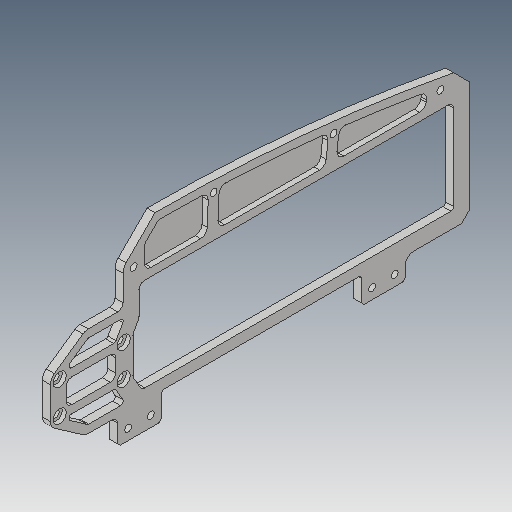
# Autodesk Inventor part: VerticalFrame
Saved by Autodesk Inventor 2019.4 (Build 234330000, 330)
## iProperties
Created: 2019-01-12
Part Number: VerticalFrame
Material: 一般
Document SubType Name: Modeling
Designer: y6tada
Density: 1 g/cm^3
Appearance: 既定
Mass: 8.8829 g
Surface Area: 108.713 cm^2
Volume: 8.8829 cm^3
Author: y6tada
Autodesk Inventor part; units mm, degrees
ref_plane "YZ Plane" through (0, 0, 0) normal (1, 0, 0) x (0, 1, 0)
ref_plane "XZ Plane" through (0, 0, 0) normal (0, 1, 0) x (-1, 0, 0)
ref_plane "XY Plane" through (0, 0, 0) normal (0, 0, 1) x (1, 0, 0)
sketch "スケッチ1" plane through (0, 0, 0) normal (1, 0, 0) x (0, 1, 0)
  line L0 (32.2256, 59) -> (0.2256, 59) construction
  line L1 (-0.7744, 56.7973) -> (-0.7744, -58)
  line L2 (0.2256, -59) -> (32.2256, -59)
  line L3 (34.2256, -57) -> (34.2256, 57)
  line L4 (-7, 67.0882) -> (-13.7744, 67.0882)
  line L5 (-14.7744, 66.0882) -> (-14.7744, 51.5882)
  line L6 (-13.7744, 50.5882) -> (-5.7744, 50.5882)
  line L7 (-4.7744, 49.5882) -> (-4.7744, -23.4118)
  line L8 (-5.7744, -24.4118) -> (-13.7744, -24.4118)
  line L9 (-14.7744, -25.4118) -> (-14.7744, -39.9118)
  line L10 (-13.7744, -40.9118) -> (-9.7744, -40.9118)
  line L11 (-3.7744, -65) -> (37.6795, -65)
  line L12 (18, 92.25) -> (6, 92.25)
  line L13 (0, 0) -> (34.2256, 0) construction
  line L14 (-6.7744, -62) -> (-3.7744, -65)
  line L15 (31, 65) -> (40.5687, 65)
  circle A0 centre (-10.7744, 63.0882) radius 1.3
  circle A1 centre (-10.7744, 54.5882) radius 1.3
  circle A2 centre (-10.7744, -28.4118) radius 1.3
  circle A3 centre (-10.7744, -36.9118) radius 1.3
  line L16 (-10.7744, 63.0882) -> (-10.7744, 54.5882) construction
  circle A4 centre (-10.7744, 63.0882) radius 2 construction
  circle A5 centre (-10.7744, 54.5882) radius 2 construction
  line L17 (-10.7744, -28.4118) -> (-10.7744, -36.9118) construction
  circle A6 centre (18, 88.75) radius 1.05 construction
  circle A7 centre (6, 88.75) radius 1.05 construction
  circle A8 centre (6, 64.75) radius 1.05 construction
  circle A9 centre (18, 64.75) radius 1.05 construction
  circle A10 centre (18, 88.75) radius 1.3
  circle A11 centre (6, 88.75) radius 1.3
  circle A12 centre (6, 64.75) radius 1.3
  circle A13 centre (18, 64.75) radius 1.3
  arc A14 (20.867, 90.7575) -> (18, 92.25) centre (18, 88.75) ccw
  arc A15 (6, 92.25) -> (3.133, 90.7575) centre (6, 88.75) ccw
  line L18 (-6.7744, -43.9118) -> (-6.7744, -62)
  arc A16 (-6.7744, -43.9118) -> (-9.7744, -40.9118) centre (-9.7744, -43.9118) ccw
  arc A17 (34.2256, 57) -> (32.2256, 59) centre (32.2256, 57) ccw
  arc A18 (32.2256, -59) -> (34.2256, -57) centre (32.2256, -57) ccw
  line L19 (43.3971, 63.8284) -> (54.2256, 53)
  arc A19 (43.6795, -59) -> (54.2256, 53) centre (-545.7744, 53) ccw
  line L20 (54.2256, 80.46) -> (54.2256, 17.89) construction
  arc A20 (-0.7744, -58) -> (0.2256, -59) centre (0.2256, -58) ccw
  arc A21 (43.3971, 63.8284) -> (40.5687, 65) centre (40.5687, 61) ccw
  line L21 (20.867, 90.7575) -> (28.367, 80.0464)
  line L22 (29, 78.0389) -> (29, 67)
  line L23 (3.133, 90.7575) -> (-4.367, 80.0464)
  line L24 (-5, 78.0389) -> (-5, 69.0882)
  line L25 (12, 92.25) -> (12, 64.3882) construction
  arc A22 (29, 78.0389) -> (28.367, 80.0464) centre (25.5, 78.0389) ccw
  arc A23 (-4.367, 80.0464) -> (-5, 78.0389) centre (-1.5, 78.0389) ccw
  arc A24 (29, 67) -> (31, 65) centre (31, 67) ccw
  arc A25 (-7, 67.0882) -> (-5, 69.0882) centre (-7, 69.0882) ccw
  line L26 (14.5, 86.25) -> (9.5, 86.25)
  line L27 (7.5, 84.25) -> (7.5, 69.75)
  line L28 (9.5, 67.75) -> (14.5, 67.75)
  line L29 (16.5, 69.75) -> (16.5, 84.25)
  arc A26 (16.5, 84.25) -> (14.5, 86.25) centre (14.5, 84.25) ccw
  arc A27 (14.5, 67.75) -> (16.5, 69.75) centre (14.5, 69.75) ccw
  arc A28 (7.5, 69.75) -> (9.5, 67.75) centre (9.5, 69.75) ccw
  arc A29 (9.5, 86.25) -> (7.5, 84.25) centre (9.5, 84.25) ccw
  line L30 (19.5, 84.3079) -> (19.5, 68.5028)
  line L31 (20, 67.6368) -> (24.5, 65.0387)
  line L32 (26, 65.9047) -> (26, 77.8812)
  line L33 (25.8192, 78.4548) -> (21.3192, 84.8815)
  arc A30 (24.5, 65.0387) -> (26, 65.9047) centre (25, 65.9047) ccw
  arc A31 (19.5, 68.5028) -> (20, 67.6368) centre (20.5, 68.5028) ccw
  arc A32 (21.3192, 84.8815) -> (19.5, 84.3079) centre (20.5, 84.3079) ccw
  arc A33 (26, 77.8812) -> (25.8192, 78.4548) centre (25, 77.8812) ccw
  line L34 (4.5, 84.3079) -> (4.5, 68.5028)
  line L35 (4, 67.6368) -> (-0.5, 65.0387)
  line L36 (-2, 65.9047) -> (-2, 77.8812)
  line L37 (-1.8192, 78.4548) -> (2.6808, 84.8815)
  arc A34 (-2, 65.9047) -> (-0.5, 65.0387) centre (-1, 65.9047) ccw
  arc A35 (4, 67.6368) -> (4.5, 68.5028) centre (3.5, 68.5028) ccw
  arc A36 (4.5, 84.3079) -> (2.6808, 84.8815) centre (3.5, 84.3079) ccw
  arc A37 (-1.8192, 78.4548) -> (-2, 77.8812) centre (-1, 77.8812) ccw
  arc A38 (-4.7744, 49.5882) -> (-5.7744, 50.5882) centre (-5.7744, 49.5882) ccw
  arc A39 (-5.7744, -24.4118) -> (-4.7744, -23.4118) centre (-5.7744, -23.4118) ccw
  line L38 (-13.7744, 67.0882) -> (-14.7744, 66.0882)
  line L39 (-14.7744, 51.5882) -> (-13.7744, 50.5882)
  line L40 (-13.7744, -24.4118) -> (-14.7744, -25.4118)
  line L41 (-14.7744, -39.9118) -> (-13.7744, -40.9118)
  circle A40 centre (40.5687, 61) radius 1.3
  line L42 (54.2256, 53) -> (-545.7744, 53) construction
  line L43 (37.6795, -65) -> (43.6795, -59)
  arc A41 (39.7277, -58.3699) -> (50.2221, 55.0291) centre (-545.7744, 53) ccw construction
  circle A42 centre (49.8194, 31) radius 1.3
  circle A43 centre (46.4476, -14) radius 1.3
  circle A44 centre (40.542, -54) radius 1.3
  line L44 (22.4952, 59.2679) -> (19.5263, 60.9821)
  line L45 (18.5263, 61.25) -> (5.4737, 61.25)
  line L46 (4.4737, 60.9821) -> (0.2256, 58.5294)
  line L47 (32.2256, 59) -> (23.4952, 59)
  arc A45 (22.4952, 59.2679) -> (23.4952, 59) centre (23.4952, 61) ccw
  arc A46 (19.5263, 60.9821) -> (18.5263, 61.25) centre (18.5263, 59.25) ccw
  arc A47 (5.4737, 61.25) -> (4.4737, 60.9821) centre (5.4737, 59.25) ccw
  arc A48 (0.2256, 58.5294) -> (-0.7744, 56.7973) centre (1.2256, 56.7973) ccw
  point P0 (34.2256, 59)
  point P1 (-0.7744, -59)
  point P2 (-0.7744, 59)
  point P3 (34.2256, -59)
  point P4 (-10.0245, 67.0882)
  point P5 (-14.7744, 67.0882)
  point P6 (-14.7744, 50.5882)
  point P7 (-4.7744, 50.5882)
  point P8 (-4.7744, -24.4118)
  point P9 (-14.7744, -24.4118)
  point P10 (-14.7744, -40.9118)
  point P11 (-4.7744, -40.9118)
  point P12 (2.5, 68.5585)
  point P13 (42.2256, 65)
  point P14 (24.5, 65)
  point P15 (-0.5, 67.0882)
  point P16 (-0.7744, 58)
  point P17 (-1.5, 78.0389)
  point P18 (22.9593, 59)
  dimension "d2" = 118
  dimension "d4" = 108
  dimension "d5" = 16.5
  dimension "d6" = 16.5
  dimension "d7" = 4
  dimension "d8" = 2.6
  dimension "d10" = 4
  dimension "d11" = 4
  dimension "d12" = 4
  dimension "d13" = 4
  dimension "d14" = 4
  dimension "d15" = 4
  dimension "d16" = 10
  dimension "d17" = 2.6
  dimension "d18" = 3.5
  dimension "d20" = 35
  dimension "d21" = 3
  dimension "d22" = 6
  dimension "d24" = 2
  dimension "d26" = 45
  dimension "d27" = 600
  dimension "d28" = 20
  dimension "d29" = 6
  dimension "d30" = 45
  dimension "d32" = 3
  dimension "d33" = 1
  dimension "d36" = 4
  dimension "d37" = 35
  dimension "d38" = 35
  dimension "d39" = 34
  dimension "d40" = 3.5
  dimension "d41" = 2
  dimension "d42" = 6
  dimension "d43" = 3
  dimension "d44" = 9
  dimension "d45" = 2
  dimension "d46" = 1
  dimension "d47" = 3
  dimension "d48" = 3
  dimension "d49" = 3
  dimension "d50" = 3.5
  dimension "d51" = 1
  dimension "d52" = 1
  dimension "d53" = 45
  dimension "d54" = 1
  dimension "d55" = 45
  dimension "d56" = 1
  dimension "d57" = 45
  dimension "d58" = 1
  dimension "d59" = 45
  dimension "d60" = 45
  dimension "d61" = 6
  dimension "d62" = 4
  dimension "d63" = 30
  dimension "d64" = 45
  dimension "d65" = 40
  dimension "d69" = 120
  dimension "d70" = 6
  dimension "d71" = 6.5
  dimension "d72" = 6
  dimension "d73" = 6
  dimension "d74" = 2
  dimension "d93" = 12
  constraints: 96 end point, 65 point on circle, 51 tangent, 43 centre point, 31 point on line, 24 equal radius, 13 symmetric about line, 10 parallel, 9 perpendicular, 7 vertical, 6 horizontal, 5 coincident, 3 concentric, 2 collinear, 2 midpoint, 6 other
  measures "d2" distance of point (34.226, -59) point (34.226, 59)
  measures "d4" distance between parallel lines of L4 L10
  measures "d5" distance of point (-14.774, -24.412) point (-14.774, -40.912)
  measures "d6" distance of point (-14.774, 67.088) point (-14.774, 50.588)
  measures "d7" distance from line of L17.start L8
  measures "d8" diameter of A2
  measures "d10" distance from line of L10 L17.end
  measures "d11" distance between parallel lines of L5 L16
  measures "d12" distance from line of L6 L16.end
  measures "d13" distance from line of L4 L16.start
  measures "d14" distance between parallel lines of L17 L9
  measures "d15" distance between parallel lines of L1 L7
  measures "d16" distance of point (-14.774, 50.588) point (-4.774, 50.588)
  measures "d17" diameter of A10
  measures "d18" radius of A14
  measures "d20" distance of point (34.226, 59) point (-0.774, 59)
  measures "d21" radius of A16
  measures "d22" distance between parallel lines of L18 L1
  measures "d24" radius of A17
  measures "d26" angle of L19 L15
  measures "d27" radius of A19
  measures "d28" distance between parallel lines of L3 L20
  measures "d29" distance between parallel lines of L11 L2
  measures "d30" angle of L14 L18
  measures "d32" distance from line of L14.start L11
  measures "d33" radius of A20
  measures "d36" radius of A21
  measures "d37" angle of L22 L21
  measures "d38" angle of L24 L23
  measures "d39" distance between parallel lines of L24 L22
  measures "d40" radius of A22
  measures "d41" radius of A24
  measures "d42" distance between parallel lines of L26 L12
  measures "d43" distance from line of A9.centre L28
  measures "d44" distance between parallel lines of L27 L29
  measures "d45" radius of A26
  measures "d46" radius of A30
  measures "d47" distance between parallel lines of L22 L32
  measures "d48" distance between parallel lines of L21 L33
  measures "d49" distance between parallel lines of L29 L30
  measures "d50" distance from line of A9.centre L31
  measures "d51" radius of A38
  measures "d52" distance of L4.end point (-14.774, 67.088)
  measures "d53" angle of L4 L38
  measures "d54" distance of L5.end point (-14.774, 50.588)
  measures "d55" angle of L5 L39
  measures "d56" distance of L8.end point (-14.774, -24.412)
  measures "d57" angle of L8 L40
  measures "d58" distance of L9.end point (-14.774, -40.912)
  measures "d59" angle of L9 L41
  measures "d60" angle of L43 L11
  measures "d61" distance from line of L43.end L11
  measures "d62" radial gap between concentric circles of A41 A19
  measures "d63" vertical distance of A42.centre A21.centre
  measures "d64" vertical distance of A43.centre A42.centre
  measures "d65" vertical distance of A44.centre A43.centre
  measures "d69" angle of L30 L31
  measures "d70" distance between parallel lines of L0 L15
  measures "d71" distance between parallel lines of L28 L45
  measures "d72" distance between parallel lines of L31 L44
  measures "d73" distance between parallel lines of L35 L46
  measures "d74" radius of A45
  measures "d93" distance between parallel lines of L42 L15
extrude "押し出し1" add sketch "スケッチ1" along normal blind 3
sketch "スケッチ2" plane through (3, 0, 0) normal (1, 0, 0) x (0, 0, -1)
  circle A0 centre (-88.75, 18) radius 1.3 projected
  circle A1 centre (-88.75, 18) radius 2.5
  circle A2 centre (-88.75, 6) radius 1.3 projected
  circle A3 centre (-88.75, 6) radius 2.5
  circle A4 centre (-64.75, 6) radius 1.3 projected
  circle A5 centre (-64.75, 6) radius 2.5
  circle A6 centre (-64.75, 18) radius 1.3 projected
  circle A7 centre (-64.75, 18) radius 2.5
  point P0 (0, 0)
  dimension "d66" = 5
  constraints: 4 centre point, 4 coincident, 3 equal radius
  measures "d66" diameter of A1
extrude "押し出し2" cut sketch "スケッチ2" against normal blind 1.5
sketch "スケッチ3" plane through (3, 0, 0) normal (1, 0, 0) x (0, 0, -1)
  circle A0 centre (-31, 49.8194) radius 1.3 construction
  line L0 (-31, 49.8194) -> (-31.9952, 22.8769) construction
  circle A1 centre (14, 46.4476) radius 1.3 construction
  line L1 (14, 46.4476) -> (11.2386, 22.0394) construction
  arc A2 (11.2386, 22.0394) -> (11.2386, 22.0394) centre (23.9128, 20.6055) ccw
  line L2 (-53, 54.2256) -> (-63.8284, 43.3971) construction
  arc A3 (59, 43.6795) -> (-53, 54.2256) centre (-53, -545.7744) ccw construction
  line L3 (-57, 34.2256) -> (57, 34.2256) construction
  line L4 (-52.4939, 50.489) -> (-56.2678, 46.7152)
  line L5 (-33.0546, 48.3772) -> (-33.3776, 39.6333)
  line L6 (-29.0574, 48.2296) -> (-29.3681, 39.8178)
  line L7 (-57, 39.7256) -> (-57, 44.9474)
  line L8 (11.8421, 45.1651) -> (11.195, 39.4445)
  line L9 (15.8168, 44.7154) -> (15.2841, 40.0066)
  circle A4 centre (54, 40.542) radius 1.3 construction
  line L10 (54, 40.542) -> (51.075, 24.5141) construction
  line L11 (48.8034, 39.9175) -> (48.6865, 39.2767)
  line L12 (-54.5, 37.2256) -> (-35.8759, 37.2256)
  line L13 (-26.8698, 37.2256) -> (8.7108, 37.2256)
  line L14 (17.7682, 37.2256) -> (46.2271, 37.2256)
  arc A5 (-35.4796, 50.9684) -> (-50.7166, 51.2212) centre (-53, -545.7744) ccw
  arc A6 (-50.7166, 51.2212) -> (-52.4939, 50.489) centre (-50.7262, 48.7212) ccw
  arc A7 (-33.0546, 48.3772) -> (-35.4796, 50.9684) centre (-35.5529, 48.4695) ccw
  arc A8 (-35.8759, 37.2256) -> (-33.3776, 39.6333) centre (-35.8759, 39.7256) ccw
  arc A9 (-57, 39.7256) -> (-54.5, 37.2256) centre (-54.5, 39.7256) ccw
  arc A10 (-56.2678, 46.7152) -> (-57, 44.9474) centre (-54.5, 44.9474) ccw
  arc A11 (9.6202, 47.9323) -> (-26.4479, 50.6348) centre (-53, -545.7744) ccw
  arc A12 (-26.4479, 50.6348) -> (-29.0574, 48.2296) centre (-26.5591, 48.1373) ccw
  arc A13 (11.8421, 45.1651) -> (9.6202, 47.9323) centre (9.358, 45.4461) ccw
  arc A14 (8.7108, 37.2256) -> (11.195, 39.4445) centre (8.7108, 39.7256) ccw
  arc A15 (-29.3681, 39.8178) -> (-26.8698, 37.2256) centre (-26.8698, 39.7256) ccw
  arc A16 (46.7618, 42.8312) -> (18.6008, 46.9163) centre (-53, -545.7744) ccw
  arc A17 (18.6008, 46.9163) -> (15.8168, 44.7154) centre (18.3009, 44.4344) ccw
  arc A18 (48.8034, 39.9175) -> (46.7618, 42.8312) centre (46.3441, 40.3663) ccw
  arc A19 (46.2271, 37.2256) -> (48.6865, 39.2767) centre (46.2271, 39.7256) ccw
  arc A20 (15.2841, 40.0066) -> (17.7682, 37.2256) centre (17.7682, 39.7256) ccw
  circle A21 centre (-61, 40.5687) radius 1.3 construction
  point P0 (0, 0)
  point P1 (-33.5774, 34.2256)
  point P2 (-29.5746, 34.2256)
  point P3 (10.6045, 34.2256)
  point P4 (14.63, 34.2256)
  point P5 (49.257, 42.4028)
  dimension "d51" = 1
  dimension "d76" = 3
  dimension "d78" = 2
  dimension "d79" = 2
  dimension "d80" = 2
  dimension "d81" = 2
  dimension "d82" = 2.5
  dimension "d83" = 3
  dimension "d84" = 2.5
  dimension "d85" = 3
  dimension "d86" = 2.5
  dimension "d87" = 3
  dimension "d88" = 3
  dimension "d89" = 4
  dimension "d90" = 5
  constraints: 35 point on circle, 27 tangent, 26 end point, 17 centre point, 13 point on line, 10 equal radius, 9 parallel, 2 collinear, 1 vertical
  measures "d76" distance between parallel lines of L2 L4
  measures "d78" distance between parallel lines of L0 L5
  measures "d79" distance between parallel lines of L6 L0
  measures "d80" distance between parallel lines of L1 L8
  measures "d81" distance between parallel lines of L1 L9
  measures "d82" radius of A6
  measures "d83" radial gap between concentric circles of A3 A11
  measures "d84" radius of A12
  measures "d85" radial gap between concentric circles of A3 A16
  measures "d86" radius of A17
  measures "d87" distance between parallel lines of L12 L3
  measures "d88" radial gap between concentric circles of A3 A5
  measures "d89" distance from line of L7 A21.centre
  measures "d90" distance between parallel lines of L10 L11
extrude "押し出し3" cut sketch "スケッチ3" against normal blind 2 contours A6 A5 A7 L5 A8 L12 A9 L7 A10 L4 | A12 A11 A13 L8 A14 L13 A15 L6 | A17 A16 A18 L11 A19 L14 A20 L9
